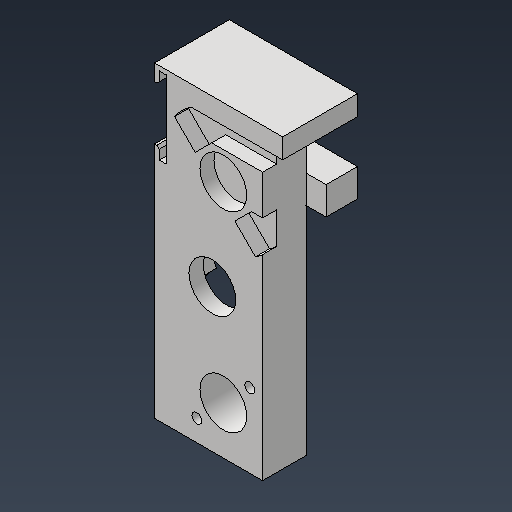
# Autodesk Inventor part: LeftGearbox
Saved by Autodesk Inventor 2026.2 (Build 302298010, 298A)
## iProperties
Created: 2026-04-13
Part Number: LeftGearbox
Material: Generic
Document SubType Name: Modeling
Designer: szymo
Density: 1 g/cm^3
Appearance: Default
Author: szymo
Autodesk Inventor part; units mm, degrees
ref_plane "YZ Plane" through (0, 0, 0) normal (1, 0, 0) x (0, 1, 0)
ref_plane "XZ Plane" through (0, 0, 0) normal (0, 1, 0) x (-1, 0, 0)
ref_plane "XY Plane" through (0, 0, 0) normal (0, 0, 1) x (1, 0, 0)
sketch "Sketch1" plane through (0, 0, 0) normal (0, 0, 1) x (1, 0, 0)
  circle A0 centre (14.7, -55.6371) radius 14.7 construction
  circle A1 centre (14.7, -55.6371) radius 14 construction
  circle A2 centre (14.7, -55.6371) radius 5
  circle A3 centre (14.7, -14.7) radius 5
  circle A4 centre (14.7, -14.7) radius 14 construction
  circle A5 centre (14.7, -14.7) radius 14.7 construction
  circle A6 centre (12.35, -35.2722) radius 5
  circle A7 centre (9.002, -47.4193) radius 8 construction
  circle A8 centre (9.002, -47.4193) radius 4.2 construction
  circle A9 centre (12.35, -35.2722) radius 9.6 construction
  line L0 (23.1, -65.8371) -> (0, -65.8371)
  line L1 (0, -65.8371) -> (0, 0)
  line L2 (0, 0) -> (23.1, 0)
  line L3 (23.1, 0) -> (23.1, -65.8371)
  circle A10 centre (12.35, -35.2722) radius 10
  circle A11 centre (9.002, -47.4193) radius 8.4
  line L4 (29.4, -55.6371) -> (23.1, -55.6371)
  line L5 (14.7, -55.6371) -> (23.1, -55.6371) construction
  line L6 (20.7104, -17.1749) -> (25.128, -21.5925) construction
  arc A12 (21.5925, -25.128) -> (25.128, -21.5925) centre (14.7, -14.7) ccw construction
  line L7 (21.5925, -25.128) -> (17.1749, -20.7104)
  arc A13 (17.1749, -20.7104) -> (20.7104, -17.1749) centre (14.7, -14.7) ccw construction
  arc A14 (7.8075, -4.272) -> (4.272, -7.8075) centre (14.7, -14.7) ccw
  line L8 (4.272, -7.8075) -> (8.6896, -12.2251)
  arc A15 (12.2251, -8.6896) -> (8.6896, -12.2251) centre (14.7, -14.7) ccw construction
  line L9 (12.2251, -8.6896) -> (7.8075, -4.272) construction
  line L10 (7.8075, -4.272) -> (23.1, -4.272)
  line L11 (12.2251, -8.6896) -> (23.1, -8.6896)
  line L12 (12.2251, -8.6896) -> (8.6896, -12.2251)
  line L13 (21.5925, -25.128) -> (23.1, -25.128)
  line L14 (20.7104, -17.1749) -> (23.1, -17.1749)
  line L15 (20.7104, -17.1749) -> (17.1749, -20.7104)
  line L16 (23.1, -4.272) -> (27.4, -4.272)
  line L17 (27.4, -4.272) -> (27.4, 0)
  line L18 (27.4, 0) -> (23.1, 0)
  circle A16 centre (9.002, -47.4193) radius 4.6
  circle A17 centre (14.7, -55.6371) radius 14.7 projected
  circle A18 centre (14.7, -55.6371) radius 14 projected
  circle A19 centre (9.0431, -61.2939) radius 1.0564 projected
  circle A20 centre (20.3569, -49.9802) radius 1.0564 projected
  circle A21 centre (14.7, -55.6371) radius 5 projected
  circle A22 centre (14.7, -55.6371) radius 14 projected
  circle A23 centre (14.7, -14.7) radius 14.7 projected
  circle A24 centre (14.7, -14.7) radius 14 projected
  line L19 (18.8355, -20.9568) -> (21.7016, -23.8229) projected
  arc A25 (21.7016, -23.8229) -> (23.8229, -21.7016) centre (14.7, -14.7) ccw projected
  line L20 (23.8229, -21.7016) -> (20.9568, -18.8355) projected
  arc A26 (18.8355, -20.9568) -> (20.9568, -18.8355) centre (14.7, -14.7) ccw projected
  arc A27 (7.6984, -5.5771) -> (5.5771, -7.6984) centre (14.7, -14.7) ccw projected
  line L21 (5.5771, -7.6984) -> (8.4432, -10.5645) projected
  arc A28 (10.5645, -8.4432) -> (8.4432, -10.5645) centre (14.7, -14.7) ccw projected
  line L22 (10.5645, -8.4432) -> (7.6984, -5.5771) projected
  circle A29 centre (14.7, -14.7) radius 5 projected
  circle A30 centre (14.7, -14.7) radius 14 projected
  arc A31 (9.8338, -26.0078) -> (9.7739, -27.4347) centre (15.759, -26.9712) ccw projected
  arc A32 (10.3221, -25.8888) -> (9.8338, -26.0078) centre (12.35, -35.2722) ccw projected
  arc A33 (11.0317, -27.1282) -> (10.3221, -25.8888) centre (5.5043, -29.47) ccw projected
  arc A34 (11.4597, -27.0704) -> (11.0317, -27.1282) centre (12.35, -35.2722) ccw projected
  arc A35 (11.815, -25.6871) -> (11.4597, -27.0704) centre (17.4104, -27.8613) ccw projected
  arc A36 (12.3173, -25.6723) -> (11.815, -25.6871) centre (12.35, -35.2722) ccw projected
  arc A37 (12.7537, -27.0321) -> (12.3173, -25.6723) centre (6.8602, -28.1735) ccw projected
  arc A38 (13.1844, -27.0645) -> (12.7537, -27.0321) centre (12.35, -35.2722) ccw projected
  arc A39 (13.8195, -25.7853) -> (13.1844, -27.0645) centre (18.8407, -29.0754) ccw projected
  arc A40 (14.314, -25.8753) -> (13.8195, -25.7853) centre (12.35, -35.2722) ccw projected
  arc A41 (14.4581, -27.2961) -> (14.314, -25.8753) centre (8.4561, -27.1873) ccw projected
  arc A42 (14.8727, -27.4174) -> (14.4581, -27.2961) centre (12.35, -35.2722) ccw projected
  arc A43 (15.7598, -26.2982) -> (14.8727, -27.4174) centre (19.9872, -30.5603) ccw projected
  arc A44 (16.2248, -26.4889) -> (15.7598, -26.2982) centre (12.35, -35.2722) ccw projected
  arc A45 (16.0704, -27.9087) -> (16.2248, -26.4889) centre (10.2221, -26.5543) ccw projected
  arc A46 (16.4507, -28.1135) -> (16.0704, -27.9087) centre (12.35, -35.2722) ccw projected
  arc A47 (17.5511, -27.2032) -> (16.4507, -28.1135) centre (20.8, -32.2511) ccw projected
  arc A48 (17.9663, -27.4865) -> (17.5511, -27.2032) centre (12.35, -35.2722) ccw projected
  arc A49 (17.52, -28.8431) -> (17.9663, -27.4865) centre (12.0812, -26.3024) ccw projected
  arc A50 (17.8494, -29.1225) -> (17.52, -28.8431) centre (12.35, -35.2722) ccw projected
  arc A51 (19.1151, -28.4609) -> (17.8494, -29.1225) centre (21.2434, -34.074) ccw projected
  arc A52 (19.4623, -28.8243) -> (19.1151, -28.4609) centre (12.35, -35.2722) ccw projected
  arc A53 (18.7437, -30.0585) -> (19.4623, -28.8243) centre (13.952, -26.4426) ccw projected
  arc A54 (19.0078, -30.4003) -> (18.7437, -30.0585) centre (12.35, -35.2722) ccw projected
  arc A55 (20.3834, -30.0163) -> (19.0078, -30.4003) centre (21.2982, -35.9492) ccw projected
  arc A56 (20.6475, -30.4439) -> (20.3834, -30.0163) centre (12.35, -35.2722) ccw projected
  arc A57 (19.688, -31.5018) -> (20.6475, -30.4439) centre (15.7527, -26.9686) ccw projected
  arc A58 (19.8753, -31.891) -> (19.688, -31.5018) centre (12.35, -35.2722) ccw projected
  arc A59 (21.3006, -31.8014) -> (19.8753, -31.891) centre (20.9619, -37.7949) ccw projected
  arc A60 (21.47, -32.2746) -> (21.3006, -31.8014) centre (12.35, -35.2722) ccw projected
  arc A61 (20.3116, -33.1099) -> (21.47, -32.2746) centre (17.4048, -27.8575) ccw projected
  arc A62 (20.4138, -33.5295) -> (20.3116, -33.1099) centre (12.35, -35.2722) ccw projected
  arc A63 (21.8266, -33.7382) -> (20.4138, -33.5295) centre (20.2492, -39.5303) ccw projected
  arc A64 (21.8939, -34.2363) -> (21.8266, -33.7382) centre (12.35, -35.2722) ccw projected
  arc A65 (20.5872, -34.8124) -> (21.8939, -34.2363) centre (18.836, -29.0705) ccw projected
  arc A66 (20.6, -35.2441) -> (20.5872, -34.8124) centre (12.35, -35.2722) ccw projected
  arc A67 (21.9385, -35.742) -> (20.6, -35.2441) centre (19.1913, -41.0796) ccw projected
  arc A68 (21.9008, -36.2432) -> (21.9385, -35.742) centre (12.35, -35.2722) ccw projected
  arc A69 (20.5028, -36.5351) -> (21.9008, -36.2432) centre (19.9836, -30.5545) ccw projected
  arc A70 (20.4255, -36.96) -> (20.5028, -36.5351) centre (12.35, -35.2722) ccw projected
  arc A71 (21.6313, -37.7253) -> (20.4255, -36.96) centre (17.8344, -42.3751) ccw projected
  arc A72 (21.4902, -38.2077) -> (21.6313, -37.7253) centre (12.35, -35.2722) ccw projected
  arc A73 (20.0621, -38.2025) -> (21.4902, -38.2077) centre (20.7977, -32.2447) ccw projected
  arc A74 (19.8981, -38.6021) -> (20.0621, -38.2025) centre (12.35, -35.2722) ccw projected
  arc A75 (20.9184, -39.6014) -> (19.8981, -38.6021) centre (16.2378, -43.3601) ccw projected
  arc A76 (20.6801, -40.0439) -> (20.9184, -39.6014) centre (12.35, -35.2722) ccw projected
  arc A77 (19.2843, -39.7419) -> (20.6801, -40.0439) centre (21.2425, -34.0672) ccw projected
  arc A78 (19.0409, -40.0987) -> (19.2843, -39.7419) centre (12.35, -35.2722) ccw projected
  arc A79 (19.8311, -41.2883) -> (19.0409, -40.0987) centre (14.4713, -43.9917) ccw projected
  arc A80 (19.506, -41.6716) -> (19.8311, -41.2883) centre (12.35, -35.2722) ccw projected
  arc A81 (18.2034, -41.086) -> (19.506, -41.6716) centre (21.2987, -35.9424) ccw projected
  arc A82 (17.8912, -41.3843) -> (18.2034, -41.086) centre (12.35, -35.2722) ccw projected
  arc A83 (18.4168, -42.7122) -> (17.8912, -41.3843) centre (12.612, -44.2422) ccw projected
  arc A84 (18.0191, -43.0195) -> (18.4168, -42.7122) centre (12.35, -35.2722) ccw projected
  arc A85 (16.8668, -42.1759) -> (18.0191, -43.0195) centre (20.9638, -37.7883) ccw projected
  arc A86 (16.4993, -42.4028) -> (16.8668, -42.1759) centre (12.35, -35.2722) ccw projected
  arc A87 (16.7374, -43.811) -> (16.4993, -42.4028) centre (10.7413, -44.1007) ccw projected
  arc A88 (16.2845, -44.0289) -> (16.7374, -43.811) centre (12.35, -35.2722) ccw projected
  arc A89 (15.3327, -42.9641) -> (16.2845, -44.0289) centre (20.2525, -39.5243) ccw projected
  arc A90 (14.9261, -43.1097) -> (15.3327, -42.9641) centre (12.35, -35.2722) ccw projected
  arc A91 (14.8662, -44.5366) -> (14.9261, -43.1097) centre (8.941, -43.5733) ccw projected
  arc A92 (14.3779, -44.6556) -> (14.8662, -44.5366) centre (12.35, -35.2722) ccw projected
  arc A93 (13.6683, -43.4162) -> (14.3779, -44.6556) centre (19.1957, -41.0744) ccw projected
  arc A94 (13.2403, -43.474) -> (13.6683, -43.4162) centre (12.35, -35.2722) ccw projected
  arc A95 (12.885, -44.8573) -> (13.2403, -43.474) centre (7.2896, -42.6831) ccw projected
  arc A96 (12.3827, -44.8722) -> (12.885, -44.8573) centre (12.35, -35.2722) ccw projected
  arc A97 (11.9463, -43.5123) -> (12.3827, -44.8722) centre (17.8398, -42.3709) ccw projected
  arc A98 (11.5156, -43.4799) -> (11.9463, -43.5123) centre (12.35, -35.2722) ccw projected
  arc A99 (10.8805, -44.7591) -> (11.5156, -43.4799) centre (5.8593, -41.469) ccw projected
  arc A100 (10.386, -44.6692) -> (10.8805, -44.7591) centre (12.35, -35.2722) ccw projected
  arc A101 (10.2419, -43.2483) -> (10.386, -44.6692) centre (16.2439, -43.3572) ccw projected
  arc A102 (9.8273, -43.1271) -> (10.2419, -43.2483) centre (12.35, -35.2722) ccw projected
  arc A103 (8.9402, -44.2462) -> (9.8273, -43.1271) centre (4.7128, -39.9841) ccw projected
  arc A104 (8.4752, -44.0555) -> (8.9402, -44.2462) centre (12.35, -35.2722) ccw projected
  arc A105 (8.6296, -42.6357) -> (8.4752, -44.0555) centre (14.4779, -43.9901) ccw projected
  arc A106 (8.2493, -42.4309) -> (8.6296, -42.6357) centre (12.35, -35.2722) ccw projected
  arc A107 (7.1489, -43.3412) -> (8.2493, -42.4309) centre (3.9, -38.2933) ccw projected
  arc A108 (6.7337, -43.0579) -> (7.1489, -43.3412) centre (12.35, -35.2722) ccw projected
  arc A109 (7.18, -41.7013) -> (6.7337, -43.0579) centre (12.6188, -44.242) ccw projected
  arc A110 (6.8506, -41.4219) -> (7.18, -41.7013) centre (12.35, -35.2722) ccw projected
  arc A111 (5.5849, -42.0835) -> (6.8506, -41.4219) centre (3.4566, -36.4704) ccw projected
  arc A112 (5.2377, -41.7201) -> (5.5849, -42.0835) centre (12.35, -35.2722) ccw projected
  arc A113 (5.9563, -40.4859) -> (5.2377, -41.7201) centre (10.748, -44.1019) ccw projected
  arc A114 (5.6922, -40.1441) -> (5.9563, -40.4859) centre (12.35, -35.2722) ccw projected
  arc A115 (4.3166, -40.5281) -> (5.6922, -40.1441) centre (3.4018, -34.5952) ccw projected
  arc A116 (4.0525, -40.1005) -> (4.3166, -40.5281) centre (12.35, -35.2722) ccw projected
  arc A117 (5.012, -39.0426) -> (4.0525, -40.1005) centre (8.9473, -43.5759) ccw projected
  arc A118 (4.8247, -38.6534) -> (5.012, -39.0426) centre (12.35, -35.2722) ccw projected
  arc A119 (3.3994, -38.743) -> (4.8247, -38.6534) centre (3.7381, -32.7495) ccw projected
  arc A120 (3.23, -38.2698) -> (3.3994, -38.743) centre (12.35, -35.2722) ccw projected
  arc A121 (4.3884, -37.4346) -> (3.23, -38.2698) centre (7.2952, -42.6869) ccw projected
  arc A122 (4.2862, -37.0149) -> (4.3884, -37.4346) centre (12.35, -35.2722) ccw projected
  arc A123 (2.8734, -36.8062) -> (4.2862, -37.0149) centre (4.4508, -31.0141) ccw projected
  arc A124 (2.8061, -36.3082) -> (2.8734, -36.8062) centre (12.35, -35.2722) ccw projected
  arc A125 (4.1128, -35.732) -> (2.8061, -36.3082) centre (5.864, -41.474) ccw projected
  arc A126 (4.1, -35.3003) -> (4.1128, -35.732) centre (12.35, -35.2722) ccw projected
  arc A127 (2.7615, -34.8024) -> (4.1, -35.3003) centre (5.5087, -29.4648) ccw projected
  arc A128 (2.7992, -34.3012) -> (2.7615, -34.8024) centre (12.35, -35.2722) ccw projected
  arc A129 (4.1972, -34.0094) -> (2.7992, -34.3012) centre (4.7164, -39.9899) ccw projected
  arc A130 (4.2745, -33.5844) -> (4.1972, -34.0094) centre (12.35, -35.2722) ccw projected
  arc A131 (3.0687, -32.8191) -> (4.2745, -33.5844) centre (6.8656, -28.1694) ccw projected
  arc A132 (3.2098, -32.3367) -> (3.0687, -32.8191) centre (12.35, -35.2722) ccw projected
  arc A133 (4.6379, -32.3419) -> (3.2098, -32.3367) centre (3.9023, -38.2997) ccw projected
  arc A134 (4.8019, -31.9423) -> (4.6379, -32.3419) centre (12.35, -35.2722) ccw projected
  arc A135 (3.7816, -30.943) -> (4.8019, -31.9423) centre (8.4622, -27.1843) ccw projected
  arc A136 (4.0199, -30.5005) -> (3.7816, -30.943) centre (12.35, -35.2722) ccw projected
  arc A137 (5.4157, -30.8025) -> (4.0199, -30.5005) centre (3.4575, -36.4772) ccw projected
  arc A138 (5.6591, -30.4457) -> (5.4157, -30.8025) centre (12.35, -35.2722) ccw projected
  arc A139 (4.8689, -29.2562) -> (5.6591, -30.4457) centre (10.2287, -26.5527) ccw projected
  arc A140 (5.194, -28.8729) -> (4.8689, -29.2562) centre (12.35, -35.2722) ccw projected
  arc A141 (6.4966, -29.4585) -> (5.194, -28.8729) centre (3.4013, -34.602) ccw projected
  arc A142 (6.8088, -29.1601) -> (6.4966, -29.4585) centre (12.35, -35.2722) ccw projected
  arc A143 (6.2832, -27.8322) -> (6.8088, -29.1601) centre (12.088, -26.3022) ccw projected
  arc A144 (6.6809, -27.5249) -> (6.2832, -27.8322) centre (12.35, -35.2722) ccw projected
  arc A145 (7.8332, -28.3685) -> (6.6809, -27.5249) centre (3.7362, -32.7561) ccw projected
  arc A146 (8.2007, -28.1416) -> (7.8332, -28.3685) centre (12.35, -35.2722) ccw projected
  arc A147 (7.9626, -26.7334) -> (8.2007, -28.1416) centre (13.9587, -26.4438) ccw projected
  arc A148 (8.4155, -26.5155) -> (7.9626, -26.7334) centre (12.35, -35.2722) ccw projected
  arc A149 (9.3673, -27.5803) -> (8.4155, -26.5155) centre (4.4475, -31.0201) ccw projected
  arc A150 (9.7739, -27.4347) -> (9.3673, -27.5803) centre (12.35, -35.2722) ccw projected
  circle A151 centre (9.002, -47.4193) radius 1.25 projected
  arc A152 (9.3068, -54.2875) -> (9.7745, -55.3819) centre (14.1081, -52.8828) ccw projected
  arc A153 (8.9469, -54.294) -> (9.3068, -54.2875) centre (9.002, -47.4193) ccw projected
  arc A154 (8.5194, -55.4047) -> (8.9469, -54.294) centre (4.0978, -53.0648) ccw projected
  arc A155 (8.1021, -55.3685) -> (8.5194, -55.4047) centre (9.002, -47.4193) ccw projected
  arc A156 (7.8722, -54.2008) -> (8.1021, -55.3685) centre (12.8606, -53.8251) ccw projected
  arc A157 (7.5188, -54.1324) -> (7.8722, -54.2008) centre (9.002, -47.4193) ccw projected
  arc A158 (6.8696, -55.1298) -> (7.5188, -54.1324) centre (3.0312, -51.9218) ccw projected
  arc A159 (6.469, -55.0077) -> (6.8696, -55.1298) centre (9.002, -47.4193) ccw projected
  arc A160 (6.4869, -53.8177) -> (6.469, -55.0077) centre (11.4444, -54.4873) ccw projected
  arc A161 (6.1555, -53.6773) -> (6.4869, -53.8177) centre (9.002, -47.4193) ccw projected
  arc A162 (5.3131, -54.518) -> (6.1555, -53.6773) centre (2.2255, -50.582) ccw projected
  arc A163 (4.9466, -54.3152) -> (5.3131, -54.518) centre (9.002, -47.4193) ccw projected
  arc A164 (5.2115, -53.155) -> (4.9466, -54.3152) centre (9.9215, -54.8407) ccw projected
  arc A165 (4.9166, -52.9487) -> (5.2115, -53.155) centre (9.002, -47.4193) ccw projected
  arc A166 (3.9178, -53.5959) -> (4.9166, -52.9487) centre (1.716, -49.104) ccw projected
  arc A167 (3.6015, -53.3214) -> (3.9178, -53.5959) centre (9.002, -47.4193) ccw projected
  arc A168 (4.1019, -52.2416) -> (3.6015, -53.3214) centre (8.3584, -54.8697) ccw projected
  arc A169 (3.8562, -51.9785) -> (4.1019, -52.2416) centre (9.002, -47.4193) ccw projected
  arc A170 (2.7447, -52.4039) -> (3.8562, -51.9785) centre (1.525, -47.5523) ccw projected
  arc A171 (2.4924, -52.0696) -> (2.7447, -52.4039) centre (9.002, -47.4193) ccw projected
  arc A172 (3.2063, -51.1174) -> (2.4924, -52.0696) centre (6.8235, -54.5731) ccw projected
  arc A173 (3.0207, -50.809) -> (3.2063, -51.1174) centre (9.002, -47.4193) ccw projected
  arc A174 (1.8451, -50.994) -> (3.0207, -50.809) centre (1.6607, -45.9949) ccw projected
  arc A175 (1.6678, -50.6146) -> (1.8451, -50.994) centre (9.002, -47.4193) ccw projected
  arc A176 (2.5641, -49.8316) -> (1.6678, -50.6146) centre (5.3837, -53.9638) ccw projected
  arc A177 (2.4467, -49.4913) -> (2.5641, -49.8316) centre (9.002, -47.4193) ccw projected
  arc A178 (1.2582, -49.4279) -> (2.4467, -49.4913) centre (2.1173, -44.4997) ccw projected
  arc A179 (1.1637, -49.0199) -> (1.2582, -49.4279) centre (9.002, -47.4193) ccw projected
  arc A180 (2.2032, -48.4404) -> (1.1637, -49.0199) centre (4.1021, -53.0685) ccw projected
  arc A181 (2.1591, -48.0831) -> (2.2032, -48.4404) centre (9.002, -47.4193) ccw projected
  arc A182 (1.0098, -47.774) -> (2.1591, -48.0831) centre (2.8747, -43.1321) ccw projected
  arc A183 (1.0022, -47.3552) -> (1.0098, -47.774) centre (9.002, -47.4193) ccw projected
  arc A184 (2.1395, -47.0045) -> (1.0022, -47.3552) centre (3.0346, -51.9263) ccw projected
  arc A185 (2.1706, -46.6459) -> (2.1395, -47.0045) centre (9.002, -47.4193) ccw projected
  arc A186 (1.1107, -46.1046) -> (2.1706, -46.6459) centre (3.9, -41.9518) ccw projected
  arc A187 (1.1904, -45.6934) -> (1.1107, -46.1046) centre (9.002, -47.4193) ccw projected
  arc A188 (2.3757, -45.5868) -> (1.1904, -45.6934) centre (2.2279, -50.5871) ccw projected
  arc A189 (2.4807, -45.2425) -> (2.3757, -45.5868) centre (9.002, -47.4193) ccw projected
  arc A190 (1.5565, -44.4926) -> (2.4807, -45.2425) centre (5.1482, -41.0105) ccw projected
  arc A191 (1.7199, -44.107) -> (1.5565, -44.4926) centre (9.002, -47.4193) ccw projected
  arc A192 (2.9015, -44.2491) -> (1.7199, -44.107) centre (1.7173, -49.1095) ccw projected
  arc A193 (3.0758, -43.9342) -> (2.9015, -44.2491) centre (9.002, -47.4193) ccw projected
  arc A194 (2.3277, -43.0086) -> (3.0758, -43.9342) centre (6.5649, -40.3493) ccw projected
  arc A195 (2.5677, -42.6653) -> (2.3277, -43.0086) centre (9.002, -47.4193) ccw projected
  arc A196 (3.6939, -43.0501) -> (2.5677, -42.6653) centre (1.5251, -47.558) ccw projected
  arc A197 (3.9298, -42.7782) -> (3.6939, -43.0501) centre (9.002, -47.4193) ccw projected
  arc A198 (3.3906, -41.7173) -> (3.9298, -42.7782) centre (8.0881, -39.9971) ccw projected
  arc A199 (3.6967, -41.4314) -> (3.3906, -41.7173) centre (9.002, -47.4193) ccw projected
  arc A200 (4.7183, -42.0419) -> (3.6967, -41.4314) centre (1.6596, -46.0004) ccw projected
  arc A201 (5.0056, -41.8251) -> (4.7183, -42.0419) centre (9.002, -47.4193) ccw projected
  arc A202 (4.6987, -40.6752) -> (5.0056, -41.8251) centre (9.6512, -39.9693) ccw projected
  arc A203 (5.0576, -40.4593) -> (4.6987, -40.6752) centre (9.002, -47.4193) ccw projected
  arc A204 (5.9299, -41.2688) -> (5.0576, -40.4593) centre (2.1151, -44.5049) ccw projected
  arc A205 (6.256, -41.1165) -> (5.9299, -41.2688) centre (9.002, -47.4193) ccw projected
  arc A206 (6.1949, -39.9279) -> (6.256, -41.1165) centre (11.1859, -40.2671) ccw projected
  arc A207 (6.5908, -39.7913) -> (6.1949, -39.9279) centre (9.002, -47.4193) ccw projected
  arc A208 (7.2758, -40.7645) -> (6.5908, -39.7913) centre (2.8715, -43.1367) ccw projected
  arc A209 (7.6264, -40.6833) -> (7.2758, -40.7645) centre (9.002, -47.4193) ccw projected
  arc A210 (7.8138, -39.508) -> (7.6264, -40.6833) centre (12.6252, -40.8775) ccw projected
  arc A211 (8.2295, -39.4566) -> (7.8138, -39.508) centre (9.002, -47.4193) ccw projected
  arc A212 (8.6971, -40.551) -> (8.2295, -39.4566) centre (3.8958, -41.9557) ccw projected
  arc A213 (9.057, -40.5445) -> (8.6971, -40.551) centre (9.002, -47.4193) ccw projected
  arc A214 (9.4846, -39.4338) -> (9.057, -40.5445) centre (13.9062, -41.7737) ccw projected
  arc A215 (9.9019, -39.47) -> (9.4846, -39.4338) centre (9.002, -47.4193) ccw projected
  arc A216 (10.1318, -40.6377) -> (9.9019, -39.47) centre (5.1434, -41.0135) ccw projected
  arc A217 (10.4851, -40.7061) -> (10.1318, -40.6377) centre (9.002, -47.4193) ccw projected
  arc A218 (11.1343, -39.7087) -> (10.4851, -40.7061) centre (14.9728, -42.9167) ccw projected
  arc A219 (11.5349, -39.8308) -> (11.1343, -39.7087) centre (9.002, -47.4193) ccw projected
  arc A220 (11.517, -41.0208) -> (11.5349, -39.8308) centre (6.5595, -40.3512) ccw projected
  arc A221 (11.8485, -41.1612) -> (11.517, -41.0208) centre (9.002, -47.4193) ccw projected
  arc A222 (12.6908, -40.3205) -> (11.8485, -41.1612) centre (15.7784, -44.2565) ccw projected
  arc A223 (13.0573, -40.5233) -> (12.6908, -40.3205) centre (9.002, -47.4193) ccw projected
  arc A224 (12.7924, -41.6836) -> (13.0573, -40.5233) centre (8.0824, -39.9978) ccw projected
  arc A225 (13.0874, -41.8898) -> (12.7924, -41.6836) centre (9.002, -47.4193) ccw projected
  arc A226 (14.0861, -41.2426) -> (13.0874, -41.8898) centre (16.2879, -45.7345) ccw projected
  arc A227 (14.4024, -41.5171) -> (14.0861, -41.2426) centre (9.002, -47.4193) ccw projected
  arc A228 (13.9021, -42.597) -> (14.4024, -41.5171) centre (9.6455, -39.9688) ccw projected
  arc A229 (14.1477, -42.86) -> (13.9021, -42.597) centre (9.002, -47.4193) ccw projected
  arc A230 (15.2592, -42.4346) -> (14.1477, -42.86) centre (16.479, -47.2862) ccw projected
  arc A231 (15.5115, -42.7689) -> (15.2592, -42.4346) centre (9.002, -47.4193) ccw projected
  arc A232 (14.7976, -43.7211) -> (15.5115, -42.7689) centre (11.1805, -40.2654) ccw projected
  arc A233 (14.9832, -44.0295) -> (14.7976, -43.7211) centre (9.002, -47.4193) ccw projected
  arc A234 (16.1589, -43.8445) -> (14.9832, -44.0295) centre (16.3432, -48.8436) ccw projected
  arc A235 (16.3361, -44.224) -> (16.1589, -43.8445) centre (9.002, -47.4193) ccw projected
  arc A236 (15.4399, -45.0069) -> (16.3361, -44.224) centre (12.6202, -40.8747) ccw projected
  arc A237 (15.5573, -45.3472) -> (15.4399, -45.0069) centre (9.002, -47.4193) ccw projected
  arc A238 (16.7457, -45.4106) -> (15.5573, -45.3472) centre (15.8867, -50.3389) ccw projected
  arc A239 (16.8402, -45.8187) -> (16.7457, -45.4106) centre (9.002, -47.4193) ccw projected
  arc A240 (15.8007, -46.3982) -> (16.8402, -45.8187) centre (13.9019, -41.77) ccw projected
  arc A241 (15.8448, -46.7554) -> (15.8007, -46.3982) centre (9.002, -47.4193) ccw projected
  arc A242 (16.9941, -47.0645) -> (15.8448, -46.7554) centre (15.1292, -51.7065) ccw projected
  arc A243 (17.0017, -47.4833) -> (16.9941, -47.0645) centre (9.002, -47.4193) ccw projected
  arc A244 (15.8644, -47.834) -> (17.0017, -47.4833) centre (14.9693, -42.9122) ccw projected
  arc A245 (15.8333, -48.1926) -> (15.8644, -47.834) centre (9.002, -47.4193) ccw projected
  arc A246 (16.8932, -48.7339) -> (15.8333, -48.1926) centre (14.1039, -52.8867) ccw projected
  arc A247 (16.8136, -49.1451) -> (16.8932, -48.7339) centre (9.002, -47.4193) ccw projected
  arc A248 (15.6283, -49.2517) -> (16.8136, -49.1451) centre (15.776, -44.2514) ccw projected
  arc A249 (15.5233, -49.596) -> (15.6283, -49.2517) centre (9.002, -47.4193) ccw projected
  arc A250 (16.4474, -50.3459) -> (15.5233, -49.596) centre (12.8557, -53.828) ccw projected
  arc A251 (16.2841, -50.7315) -> (16.4474, -50.3459) centre (9.002, -47.4193) ccw projected
  arc A252 (15.1025, -50.5894) -> (16.2841, -50.7315) centre (16.2866, -45.729) ccw projected
  arc A253 (14.9282, -50.9043) -> (15.1025, -50.5894) centre (9.002, -47.4193) ccw projected
  arc A254 (15.6762, -51.8299) -> (14.9282, -50.9043) centre (11.439, -54.4892) ccw projected
  arc A255 (15.4363, -52.1732) -> (15.6762, -51.8299) centre (9.002, -47.4193) ccw projected
  arc A256 (14.31, -51.7885) -> (15.4363, -52.1732) centre (16.4789, -47.2805) ccw projected
  arc A257 (14.0741, -52.0603) -> (14.31, -51.7885) centre (9.002, -47.4193) ccw projected
  arc A258 (14.6134, -53.1212) -> (14.0741, -52.0603) centre (9.9159, -54.8414) ccw projected
  arc A259 (14.3073, -53.4071) -> (14.6134, -53.1212) centre (9.002, -47.4193) ccw projected
  arc A260 (13.2856, -52.7966) -> (14.3073, -53.4071) centre (16.3443, -48.8381) ccw projected
  arc A261 (12.9983, -53.0134) -> (13.2856, -52.7966) centre (9.002, -47.4193) ccw projected
  arc A262 (13.3052, -54.1633) -> (12.9983, -53.0134) centre (8.3528, -54.8692) ccw projected
  arc A263 (12.9464, -54.3793) -> (13.3052, -54.1633) centre (9.002, -47.4193) ccw projected
  arc A264 (12.074, -53.5697) -> (12.9464, -54.3793) centre (15.8889, -50.3336) ccw projected
  arc A265 (11.7479, -53.7221) -> (12.074, -53.5697) centre (9.002, -47.4193) ccw projected
  arc A266 (11.809, -54.9106) -> (11.7479, -53.7221) centre (6.818, -54.5714) ccw projected
  arc A267 (11.4131, -55.0473) -> (11.809, -54.9106) centre (9.002, -47.4193) ccw projected
  arc A268 (10.7281, -54.074) -> (11.4131, -55.0473) centre (15.1325, -51.7018) ccw projected
  arc A269 (10.3775, -54.1552) -> (10.7281, -54.074) centre (9.002, -47.4193) ccw projected
  arc A270 (10.1902, -55.3305) -> (10.3775, -54.1552) centre (5.3787, -53.9611) ccw projected
  arc A271 (9.7745, -55.3819) -> (10.1902, -55.3305) centre (9.002, -47.4193) ccw projected
  circle A272 centre (9.002, -47.4193) radius 1.25 projected
  arc A273 (10.0792, -44.7807) -> (10.0684, -43.3569) centre (6.4384, -44.0965) ccw projected
  arc A274 (10.4144, -44.9439) -> (10.0792, -44.7807) centre (9.002, -47.4193) ccw projected
  arc A275 (11.5418, -44.0742) -> (10.4144, -44.9439) centre (13.1986, -47.3876) ccw projected
  arc A276 (11.9567, -44.4343) -> (11.5418, -44.0742) centre (9.002, -47.4193) ccw projected
  arc A277 (11.2542, -45.6728) -> (11.9567, -44.4343) centre (8.4432, -43.2599) ccw projected
  arc A278 (11.4629, -45.9817) -> (11.2542, -45.6728) centre (9.002, -47.4193) ccw projected
  arc A279 (12.874, -45.7923) -> (11.4629, -45.9817) centre (12.6522, -49.4902) ccw projected
  arc A280 (13.0533, -46.3116) -> (12.874, -45.7923) centre (9.002, -47.4193) ccw projected
  arc A281 (11.8257, -47.0329) -> (13.0533, -46.3116) centre (10.5978, -43.5377) ccw projected
  arc A282 (11.8519, -47.4048) -> (11.8257, -47.0329) centre (9.002, -47.4193) ccw projected
  arc A283 (13.1688, -47.9463) -> (11.8519, -47.4048) centre (11.1277, -51.0378) ccw projected
  arc A284 (13.0643, -48.4857) -> (13.1688, -47.9463) centre (9.002, -47.4193) ccw projected
  arc A285 (11.6405, -48.4965) -> (13.0643, -48.4857) centre (12.3247, -44.8557) ccw projected
  arc A286 (11.4774, -48.8317) -> (11.6405, -48.4965) centre (9.002, -47.4193) ccw projected
  arc A287 (12.347, -49.9591) -> (11.4774, -48.8317) centre (9.0336, -51.6159) ccw projected
  arc A288 (11.9869, -50.374) -> (12.347, -49.9591) centre (9.002, -47.4193) ccw projected
  arc A289 (10.7484, -49.6715) -> (11.9869, -50.374) centre (13.1614, -46.8605) ccw projected
  arc A290 (10.4395, -49.8802) -> (10.7484, -49.6715) centre (9.002, -47.4193) ccw projected
  arc A291 (10.629, -51.2913) -> (10.4395, -49.8802) centre (6.9311, -51.0695) ccw projected
  arc A292 (10.1096, -51.4706) -> (10.629, -51.2913) centre (9.002, -47.4193) ccw projected
  arc A293 (9.3883, -50.2429) -> (10.1096, -51.4706) centre (12.8835, -49.0151) ccw projected
  arc A294 (9.0165, -50.2692) -> (9.3883, -50.2429) centre (9.002, -47.4193) ccw projected
  arc A295 (8.4749, -51.5861) -> (9.0165, -50.2692) centre (5.3834, -49.545) ccw projected
  arc A296 (7.9356, -51.4816) -> (8.4749, -51.5861) centre (9.002, -47.4193) ccw projected
  arc A297 (7.9247, -50.0578) -> (7.9356, -51.4816) centre (11.5656, -50.742) ccw projected
  arc A298 (7.5895, -49.8946) -> (7.9247, -50.0578) centre (9.002, -47.4193) ccw projected
  arc A299 (6.4622, -50.7643) -> (7.5895, -49.8946) centre (4.8053, -47.4509) ccw projected
  arc A300 (6.0473, -50.4042) -> (6.4622, -50.7643) centre (9.002, -47.4193) ccw projected
  arc A301 (6.7498, -49.1657) -> (6.0473, -50.4042) centre (9.5607, -51.5786) ccw projected
  arc A302 (6.5411, -48.8568) -> (6.7498, -49.1657) centre (9.002, -47.4193) ccw projected
  arc A303 (5.1299, -49.0462) -> (6.5411, -48.8568) centre (5.3518, -45.3483) ccw projected
  arc A304 (4.9507, -48.5269) -> (5.1299, -49.0462) centre (9.002, -47.4193) ccw projected
  arc A305 (6.1783, -47.8056) -> (4.9507, -48.5269) centre (7.4062, -51.3008) ccw projected
  arc A306 (6.152, -47.4338) -> (6.1783, -47.8056) centre (9.002, -47.4193) ccw projected
  arc A307 (4.8352, -46.8922) -> (6.152, -47.4338) centre (6.8763, -43.8007) ccw projected
  arc A308 (4.9396, -46.3529) -> (4.8352, -46.8922) centre (9.002, -47.4193) ccw projected
  arc A309 (6.3634, -46.342) -> (4.9396, -46.3529) centre (5.6792, -49.9828) ccw projected
  arc A310 (6.5266, -46.0068) -> (6.3634, -46.342) centre (9.002, -47.4193) ccw projected
  arc A311 (5.6569, -44.8794) -> (6.5266, -46.0068) centre (8.9703, -43.2226) ccw projected
  arc A312 (6.0171, -44.4646) -> (5.6569, -44.8794) centre (9.002, -47.4193) ccw projected
  arc A313 (7.2555, -45.1671) -> (6.0171, -44.4646) centre (4.8426, -47.978) ccw projected
  arc A314 (7.5644, -44.9584) -> (7.2555, -45.1671) centre (9.002, -47.4193) ccw projected
  arc A315 (7.375, -43.5472) -> (7.5644, -44.9584) centre (11.0729, -43.7691) ccw projected
  arc A316 (7.8943, -43.368) -> (7.375, -43.5472) centre (9.002, -47.4193) ccw projected
  arc A317 (8.6156, -44.5956) -> (7.8943, -43.368) centre (5.1205, -45.8234) ccw projected
  arc A318 (8.9875, -44.5693) -> (8.6156, -44.5956) centre (9.002, -47.4193) ccw projected
  arc A319 (9.529, -43.2525) -> (8.9875, -44.5693) centre (12.6205, -45.2935) ccw projected
  arc A320 (10.0684, -43.3569) -> (9.529, -43.2525) centre (9.002, -47.4193) ccw projected
  circle A321 centre (12.35, -35.2722) radius 4.8 projected
  line L23 (2.5, -1) -> (1, -1)
  line L24 (1, -1) -> (1, -17.5)
  line L25 (1, -17.5) -> (2.5, -17.5)
  line L26 (2.5, -17.5) -> (2.5, -1)
  line L27 (1.5, -1) -> (1.5, -17) projected
  line L28 (2.5, -1) -> (1.5, -1) projected
  line L29 (2.5, -17) -> (2.5, -1) projected
  line L30 (2.5, -17) -> (1.5, -17) projected
  line L31 (1, -15) -> (0, -15)
  line L32 (1, -3.5) -> (0, -3.5)
  point P0 (0, 0)
  point P1 (3.9544, -40.7049)
  point P2 (16.7767, -44.2391)
  point P3 (13.2732, -40.1862)
  point P4 (9.0396, -39.0193)
  point P5 (13.0569, -45.2472)
  point P6 (6.6325, -43.4765)
  point P7 (16.5957, -51.0104)
  point P8 (9.7023, -55.79)
  point P9 (0.0031, -15)
  point P10 (0, -14.7)
  dimension "d0" = 4.5
  dimension "d2" = 0.4
  dimension "d3" = 0.4
  dimension "d5" = 6.3
  dimension "d8" = 2
  dimension "d10" = 0.4
  dimension "d19" = 10
  dimension "d20" = 1
  dimension "d21" = 1
  dimension "d22" = 1
  dimension "d24" = 1
  dimension "d25" = 1
  dimension "d26" = 1
  dimension "d27" = 1
  dimension "d28" = 1
  dimension "d56" = 0.5
  dimension "d57" = 0.5
  dimension "d77" = 2.5
  dimension "d78" = 2.5
  constraints: 50 end point, 13 centre point, 12 point on line, 11 perpendicular, 10 coincident, 8 point on circle, 5 parallel, 5 tangent, 2 horizontal, 2 horizontal alignment, 1 collinear, 17 other
  measures "d5" distance of L4.start L4.end
  measures "d8" distance edge to line of A5 L17
  measures "d19" diameter of A6
  measures "d20" distance between parallel lines of L7 L19
  measures "d21" radial gap between concentric circles of A12 A25
  measures "d22" radial gap between concentric circles of A13 A26
  measures "d24" distance between parallel lines of L6 L20
  measures "d25" distance between parallel lines of L9 L22
  measures "d26" distance between parallel lines of L8 L21
  measures "d27" radial gap between concentric circles of A28 A15
  measures "d28" radial gap between concentric circles of A14 A27
  measures "d56" distance between parallel lines of L24 L27
  measures "d57" distance between parallel lines of L25 L30
  measures "d77" distance between parallel lines of L28 L32
  measures "d78" distance between parallel lines of L25 L31
extrude "Extrusion1" add sketch "Sketch1" against normal blind 1.6 contours A2 A11 A10 A18 L3 L0 | A2 A253 A252 A251 A250 A249 A248 A247 A246 A245 A244 A243 A242 A241 A240 A239 A238 A237 A236 A10 A11 | A11 A18 A178 A177 A176 A175 A174 A173 A172 A171 A170 A169 A168 A167 A166 A165 A164 A163 A162 A161 A160 A159 A158 A157 A156 A155 A154 A153 A152 A2 | A2 A152 A153 A154 A155 A156 A157 A158 A159 A160 A161 A162 A163 A164 A165 A166 A167 A168 A169 A170 A171 A172 A173 A174 A175 A176 A177 A178 A18 A16 A10 A236 A237 A238 A239 A240 A241 A242 A243 A244 A245 A246 A247 A248 A249 A250 A251 A252 A253 | A18 L0 A17 A11 | A11 A17 A178 A18 | A11 A88 A87 A86 A85 A84 A83 A18 A10 | A10 A236 A235 A89 A88 A11 | A17 L1 L31 A23 A10 A11 | A11 A10 A201 A200 A199 A198 A197 A196 A195 A194 A193 A192 A191 A190 A189 A188 A187 A186 A185 A184 A183 A182 A17 A180 A179 A178 | A178 A17 A180 A181 A182 A10 A16 A18 | A10 A16 A96 A95 A94 A93 A92 A91 A233 A234 A89 A235 A236 | A18 A83 A82 A17 A10 | A10 A17 L3 A18 | A88 A89 A235 A234 A232 A231 A230 A229 A228 A18 A11 | A11 A18 A83 A84 A85 A86 A87 A88 | A11 A116 A115 A114 A113 A204 A203 A202 A201 A10 | A10 A23 A147 A146 A145 A144 A143 A142 A141 A140 A139 A138 A137 A136 A135 A134 A133 A132 A131 A130 A129 A128 A127 A126 A125 A124 A123 A122 A121 A120 A119 A118 A117 A116 A11 | A178 A179 A180 A17 | A17 L0 L1 | A18 A311 A310 A309 A308 A307 A306 A305 A304 A303 A302 A301 A300 A299 A298 A297 A296 A295 A294 A293 A292 A291 A290 A289 A288 A287 A286 A285 A284 A283 A282 A281 A280 A279 A278 A277 A10 A16 | A16 A10 A18 A313 A312 A311 | A10 A277 A276 A275 A99 A16 A97 A96 | A17 A82 A81 A80 A79 A78 A77 A76 A75 A74 A73 A72 A71 A70 A69 A68 A67 A66 A65 A64 A63 A62 A61 A60 A59 A58 A57 A56 A55 A54 A53 A52 A23 A10 | A10 A23 L3 A17 | A18 A11 A17 A82 A83 | A18 A228 A227 A226 A225 A224 A17 A11 | A23 L31 A24 A10 | A10 A24 A147 A23 | A201 A202 A203 A204 A113 A112 A111 A110 A109 A108 A17 A10 | A10 A17 A182 A183 A184 A185 A186 A187 A188 A189 A190 A191 A192 A193 A194 A195 A196 A197 A198 A199 A200 A201 | A116 A117 A118 A119 A120 A121 A122 A123 A124 A125 A126 A127 A128 A129 A130 A131 A132 A133 A134 A135 A136 A137 A138 A139 A140 A141 A142 A143 A144 A145 A146 A147 A23 A50 A51 A52 A53 A54 A55 A56 A57 A58 A59 A60 A61 A62 A63 A64 A65 A66 A67 A68 A69 A70 A71 A72 A73 A74 A75 A76 A77 A78 A79 A80 A81 A82 A17 A11 A6 | A11 A6 A215 A214 A213 A212 A211 A210 A209 A208 A207 A206 A205 A204 A113 A114 A115 A116 | A17 A182 A181 A180 | A16 A108 A107 A105 A18 A317 A316 A315 A10 | A10 A17 A108 A16 | A311 A312 A313 A18 | A18 A313 A314 A315 A10 A317 A318 A277 A278 A279 A280 A281 A282 A283 A284 A285 A286 A287 A288 A289 A290 A291 A292 A293 A294 A295 A296 A297 A298 A299 A300 A301 A302 A303 A304 A305 A306 A307 A308 A309 A310 A311 | A10 A318 A319 A103 A320 A273 A274 A275 A100 A99 A276 A277 | A96 A97 A16 | A16 A97 A98 A99 A18 A225 A226 A228 A229 A230 A231 A232 A89 A90 A91 A233 A92 A93 A94 A95 A96 | A89 A234 A235 | A17 A224 A223 A222 A221 A220 A6 A11 | A18 A226 A227 A228 | A24 L31 L24 L25 L26 L3 L10 A14 L8 L12 L11 L14 L15 L7 L13 A10 | A10 A24 A49 A48 A47 A46 A45 A44 A43 A42 A41 A40 A39 A38 A37 A36 A35 A34 A33 A32 A31 A150 A149 A148 A147 | A147 A24 A49 A50 A23 | A18 A315 A10 | A10 A315 A314 A313 A18 | A108 A17 A224 A225 A18 A16 A105 A106 A107 | A16 A107 A108 | A318 A317 A10 | A10 A317 A18 A105 A104 A103 A319 A318 | A16 A99 A98 A97 | A234 A233 A91 A232 A89 | A23 A52 A51 A50 A49 A24 A10 | A10 A24 L3 A23 | A17 A108 A109 A110 A111 A112 A113 A204 A205 A206 A207 A208 A209 A210 A211 A212 A213 A214 A215 A6 A216 A217 A218 A220 A221 A222 A223 A224 | A226 A225 A18 | A147 A148 A149 A150 A31 A32 A33 A34 A35 A36 A37 A38 A39 A40 A41 A42 A43 A44 A45 A46 A47 A48 A49 A24 | A23 A51 A50 | L1 L2 A23 L26 L23 L24 L32 | A315 A18 A317 A10 | A315 A316 A317 A18 | A107 A106 A105 A16 | A99 A275 A100 A101 A102 A103 A320 A319 A104 A105 A18 A16 | A232 A91 A90 A89 | A23 A51 A52 | A6 A218 A217 A216 | A16 A18 A105 | A319 A320 A103 | A99 A100 A275 | A91 A233 A232 | L13 L7 L15 L14 L3 L20 A26 L19 A25 | A23 L3 L18 L17 L16 | L16 A24 L3 A23 | L2 L3 A23 | A23 L3 A24 L26 | A103 A102 A101 A100 A275 A274 A273 A320 | A25 L19 A26 L20 L3 | L16 L3 A24 | L3 L11 L12 L8 A14 L10 | A3 | A19 | A20 | L22 A28 L21 A27 | A151 picked at (24.5137, -4.0777)
extrude "Extrusion2" add sketch "Sketch1" against normal blind 3.1 contours A2 A11 A10 A18 L3 L0 | A2 A253 A252 A251 A250 A249 A248 A247 A246 A245 A244 A243 A242 A241 A240 A239 A238 A237 A236 A10 A11 | A11 A18 A178 A177 A176 A175 A174 A173 A172 A171 A170 A169 A168 A167 A166 A165 A164 A163 A162 A161 A160 A159 A158 A157 A156 A155 A154 A153 A152 A2 | A2 A152 A153 A154 A155 A156 A157 A158 A159 A160 A161 A162 A163 A164 A165 A166 A167 A168 A169 A170 A171 A172 A173 A174 A175 A176 A177 A178 A18 A16 A10 A236 A237 A238 A239 A240 A241 A242 A243 A244 A245 A246 A247 A248 A249 A250 A251 A252 A253 | A18 L0 A17 A11 | A11 A17 A178 A18 | A11 A88 A87 A86 A85 A84 A83 A18 A10 | A10 A236 A235 A89 A88 A11 | A17 L1 L31 A23 A10 A11 | A11 A10 A201 A200 A199 A198 A197 A196 A195 A194 A193 A192 A191 A190 A189 A188 A187 A186 A185 A184 A183 A182 A17 A180 A179 A178 | A178 A17 A180 A181 A182 A10 A16 A18 | A10 A16 A96 A95 A94 A93 A92 A91 A233 A234 A89 A235 A236 | A18 A83 A82 A17 A10 | A10 A17 L3 A18 | A88 A89 A235 A234 A232 A231 A230 A229 A228 A18 A11 | A11 A18 A83 A84 A85 A86 A87 A88 | A11 A116 A115 A114 A113 A204 A203 A202 A201 A10 | A10 A23 A147 A146 A145 A144 A143 A142 A141 A140 A139 A138 A137 A136 A135 A134 A133 A132 A131 A130 A129 A128 A127 A126 A125 A124 A123 A122 A121 A120 A119 A118 A117 A116 A11 | A178 A179 A180 A17 | A17 L0 L1 | A17 A82 A81 A80 A79 A78 A77 A76 A75 A74 A73 A72 A71 A70 A69 A68 A67 A66 A65 A64 A63 A62 A61 A60 A59 A58 A57 A56 A55 A54 A53 A52 A23 A10 | A10 A23 L3 A17 | A18 A11 A17 A82 A83 | A18 A228 A227 A226 A225 A224 A17 A11 | A23 L31 A24 A10 | A10 A24 A147 A23 | A201 A202 A203 A204 A113 A112 A111 A110 A109 A108 A17 A10 | A10 A17 A182 A183 A184 A185 A186 A187 A188 A189 A190 A191 A192 A193 A194 A195 A196 A197 A198 A199 A200 A201 | A116 A117 A118 A119 A120 A121 A122 A123 A124 A125 A126 A127 A128 A129 A130 A131 A132 A133 A134 A135 A136 A137 A138 A139 A140 A141 A142 A143 A144 A145 A146 A147 A23 A50 A51 A52 A53 A54 A55 A56 A57 A58 A59 A60 A61 A62 A63 A64 A65 A66 A67 A68 A69 A70 A71 A72 A73 A74 A75 A76 A77 A78 A79 A80 A81 A82 A17 A11 A6 | A11 A6 A215 A214 A213 A212 A211 A210 A209 A208 A207 A206 A205 A204 A113 A114 A115 A116 | A17 A182 A181 A180 | A10 A17 A108 A16 | A16 A97 A98 A99 A18 A225 A226 A228 A229 A230 A231 A232 A89 A90 A91 A233 A92 A93 A94 A95 A96 | A89 A234 A235 | A17 A224 A223 A222 A221 A220 A6 A11 | A18 A226 A227 A228 | A24 L31 L24 L25 L26 L3 L10 A14 L8 L12 L11 L14 L15 L7 L13 A10 | A10 A24 A49 A48 A47 A46 A45 A44 A43 A42 A41 A40 A39 A38 A37 A36 A35 A34 A33 A32 A31 A150 A149 A148 A147 | A147 A24 A49 A50 A23 | A108 A17 A224 A225 A18 A16 A105 A106 A107 | A16 A99 A98 A97 | A234 A233 A91 A232 A89 | A23 A52 A51 A50 A49 A24 A10 | A10 A24 L3 A23 | A17 A108 A109 A110 A111 A112 A113 A204 A205 A206 A207 A208 A209 A210 A211 A212 A213 A214 A215 A6 A216 A217 A218 A220 A221 A222 A223 A224 | A226 A225 A18 | A147 A148 A149 A150 A31 A32 A33 A34 A35 A36 A37 A38 A39 A40 A41 A42 A43 A44 A45 A46 A47 A48 A49 A24 | A23 A51 A50 | L1 L2 A23 L26 L23 L24 L32 | A107 A106 A105 A16 | A232 A91 A90 A89 | A23 A51 A52 | A6 A218 A217 A216 | A91 A233 A232 | L13 L7 L15 L14 L3 L20 A26 L19 A25 | A23 L3 L18 L17 L16 | L16 A24 L3 A23 | L2 L3 A23 | A23 L3 A24 L26 | A25 L19 A26 L20 L3 | L16 L3 A24 | L3 L11 L12 L8 A14 L10 | A3 | A19 | A20 | L22 A28 L21 A27 picked at (24.5137, -4.0777)
extrude "Extrusion3" add sketch "Sketch1" against normal blind 6.2 contours A2 A11 A10 A18 L3 L0 | A2 A253 A252 A251 A250 A249 A248 A247 A246 A245 A244 A243 A242 A241 A240 A239 A238 A237 A236 A10 A11 | A11 A18 A178 A177 A176 A175 A174 A173 A172 A171 A170 A169 A168 A167 A166 A165 A164 A163 A162 A161 A160 A159 A158 A157 A156 A155 A154 A153 A152 A2 | A2 A152 A153 A154 A155 A156 A157 A158 A159 A160 A161 A162 A163 A164 A165 A166 A167 A168 A169 A170 A171 A172 A173 A174 A175 A176 A177 A178 A18 A16 A10 A236 A237 A238 A239 A240 A241 A242 A243 A244 A245 A246 A247 A248 A249 A250 A251 A252 A253 | A18 L0 A17 A11 | A11 A17 A178 A18 | A17 L1 L31 A23 A10 A11 | A11 A10 A201 A200 A199 A198 A197 A196 A195 A194 A193 A192 A191 A190 A189 A188 A187 A186 A185 A184 A183 A182 A17 A180 A179 A178 | A178 A17 A180 A181 A182 A10 A16 A18 | A10 A17 L3 A18 | A178 A179 A180 A17 | A17 L0 L1 | A10 A23 L3 A17 | A23 L31 A24 A10 | A10 A17 A182 A183 A184 A185 A186 A187 A188 A189 A190 A191 A192 A193 A194 A195 A196 A197 A198 A199 A200 A201 | A17 A182 A181 A180 | A24 L31 L24 L25 L26 L3 L10 A14 L8 L12 L11 L14 L15 L7 L13 A10 | A10 A24 L3 A23 | L1 L2 A23 L26 L23 L24 L32 | L13 L7 L15 L14 L3 L20 A26 L19 A25 | A23 L3 L18 L17 L16 | L16 A24 L3 A23 | L2 L3 A23 | A23 L3 A24 L26 | A25 L19 A26 L20 L3 | L16 L3 A24 | L3 L11 L12 L8 A14 L10 | A3 | A19 | A20 | L22 A28 L21 A27 picked at (24.5137, -4.0777)
ref_plane "Work Plane1" through (6.5814, -41.0408, -9.3) normal (0, 0, -1) x (0.0707652, 0.997493, 0)
extrude "Extrusion4" add sketch "Sketch1" against normal up to surface (9.3 mm away) contours A2 A11 A10 A18 L3 L0 | A18 L0 A17 A11 | A17 L1 L31 A23 A10 A11 | A10 A17 L3 A18 | A17 L0 L1 | A10 A23 L3 A17 | A23 L31 A24 A10 | A24 L31 L24 L25 L26 L3 L10 A14 L8 L12 L11 L14 L15 L7 L13 A10 | A10 A24 L3 A23 | L1 L2 A23 L26 L23 L24 L32 | L13 L7 L15 L14 L3 L20 A26 L19 A25 | A23 L3 L18 L17 L16 | L16 A24 L3 A23 | L2 L3 A23 | A23 L3 A24 L26 | A25 L19 A26 L20 L3 | L16 L3 A24 | L3 L11 L12 L8 A14 L10 | A3 | A19 | A20 | L22 A28 L21 A27 picked at (24.5137, -4.0777)
sketch "Sketch2" plane through (0, 0, 0) normal (0, 0, 1) x (1, 0, 0)
  line L0 (23.1, 0) -> (0, 0)
  line L1 (0, 0) -> (0, -29.4)
  line L2 (0, -29.4) -> (23.1, -29.4)
  line L3 (23.1, -29.4) -> (23.1, 0)
  arc A0 (7.8075, -4.272) -> (4.272, -7.8075) centre (14.7, -14.7) ccw
  line L4 (4.272, -7.8075) -> (8.6896, -12.2251)
  arc A1 (12.2251, -8.6896) -> (8.6896, -12.2251) centre (14.7, -14.7) ccw construction
  line L5 (12.2251, -8.6896) -> (7.8075, -4.272)
  line L6 (20.7104, -17.1749) -> (25.128, -21.5925)
  arc A2 (21.5925, -25.128) -> (25.128, -21.5925) centre (14.7, -14.7) ccw
  line L7 (21.5925, -25.128) -> (17.1749, -20.7104)
  line L8 (7.8075, -4.272) -> (23.1, -4.272)
  line L9 (12.2251, -8.6896) -> (8.6896, -12.2251)
  line L10 (12.2251, -8.6896) -> (23.1, -8.6896)
  line L11 (20.7104, -17.1749) -> (23.1, -17.1749)
  line L12 (20.7104, -17.1749) -> (17.1749, -20.7104)
  line L13 (21.5925, -25.128) -> (23.1, -25.128)
  line L14 (18.8355, -20.9568) -> (21.7016, -23.8229) projected
  arc A3 (21.7016, -23.8229) -> (23.8229, -21.7016) centre (14.7, -14.7) ccw projected
  line L15 (23.8229, -21.7016) -> (20.9568, -18.8355) projected
  arc A4 (18.8355, -20.9568) -> (20.9568, -18.8355) centre (14.7, -14.7) ccw projected
  arc A5 (7.6984, -5.5771) -> (5.5771, -7.6984) centre (14.7, -14.7) ccw projected
  line L16 (5.5771, -7.6984) -> (8.4432, -10.5645) projected
  arc A6 (10.5645, -8.4432) -> (8.4432, -10.5645) centre (14.7, -14.7) ccw projected
  line L17 (10.5645, -8.4432) -> (7.6984, -5.5771) projected
  circle A7 centre (14.7, -14.7) radius 5 projected
  circle A8 centre (14.7, -14.7) radius 14 projected
  circle A9 centre (14.7, -14.7) radius 14.7 projected
  circle A10 centre (14.7, -14.7) radius 14 projected
  circle A11 centre (14.7, -14.7) radius 5
  arc A12 (17.1749, -20.7104) -> (20.7104, -17.1749) centre (14.7, -14.7) ccw construction
  point P0 (0, 0)
  point P1 (23.1, -23.9569)
  point P2 (23.1, -19.5645)
  point P3 (20.0033, -20.0033)
  dimension "d34" = 6.3
  dimension "d35" = 1
  dimension "d36" = 1
  dimension "d39" = 1
  dimension "d41" = 1
  dimension "d50" = 1
  dimension "d51" = 1
  dimension "d53" = 1
  dimension "d55" = 1
  constraints: 28 end point, 9 point on circle, 5 centre point, 5 coincident, 5 perpendicular, 5 point on line, 4 tangent, 3 parallel, 1 horizontal
  measures "d34" distance edge to line of A9 L3
  measures "d35" distance between parallel lines of L4 L16
  measures "d36" distance between parallel lines of L5 L17
  measures "d39" distance between parallel lines of L7 L14
  measures "d41" distance between parallel lines of L6 L15
  measures "d50" radial gap between concentric circles of A1 A6
  measures "d51" radial gap between concentric circles of A5 A0
  measures "d53" radial gap between concentric circles of A3 A2
  measures "d55" radial gap between concentric circles of A4 A12
extrude "Extrusion5" cut sketch "Sketch2" against normal blind 3 contours L3 L10 L5 L8 | L5 L9 L4 A0 | L3 L6 L11 | A2 L7 L12 L6 L3 L15 A4 L14 A3 | A3 L14 A4 L15 L3 | L17 A6 L16 A5 | A7
sketch "Sketch3" plane through (27.4, 0, -9.3) normal (0, 0, -1) x (-1, 0, 0)
  circle A0 centre (18.3569, -61.2939) radius 1.0564
  circle A1 centre (7.0431, -49.9802) radius 1.0564
  circle A2 centre (12.7, -55.6371) radius 14.7
  circle A3 centre (12.7, -14.7) radius 14.7
  line L0 (4.3, -65.8371) -> (27.4, -65.8371)
  line L1 (27.4, -65.8371) -> (27.4, 0)
  line L2 (27.4, 0) -> (4.3, 0)
  line L3 (0, -4.272) -> (0, 0)
  line L4 (0, -4.272) -> (0, 0) projected
  line L5 (0, 0) -> (27.4, 0) projected
  line L6 (4.3, 0) -> (0, 0)
  line L7 (25.9, -1) -> (25.9, -17)
  line L8 (24.9, -1) -> (25.9, -1)
  line L9 (24.9, -17) -> (24.9, -1)
  line L10 (24.9, -17) -> (25.9, -17)
  line L11 (27.4, -19.5) -> (4.3, -19.5)
  line L12 (4.3, -19.5) -> (4.3, -23.9569)
  line L13 (4.3, -19.5) -> (0, -19.5)
  line L14 (0, -19.5) -> (0, -4.272) construction
  line L15 (0, -19.5) -> (0, -13.5)
  line L16 (0, -13.5) -> (24.4, -13.5)
  line L17 (24.4, -13.5) -> (24.4, -17.5)
  line L18 (24.4, -17.5) -> (26.4, -17.5)
  line L19 (26.4, -17.5) -> (26.4, -15)
  line L20 (26.4, -15) -> (27.4, -15)
  line L21 (27.4, -3.5) -> (26.4, -3.5)
  line L22 (26.4, -3.5) -> (26.4, -1)
  line L23 (26.4, -1) -> (24.4, -1)
  line L24 (24.4, -1) -> (24.4, -4.272)
  line L25 (4.3, -4.272) -> (0, -4.272) projected
  line L26 (24.4, -4.272) -> (0, -4.272)
  circle A4 centre (7.0431, -49.9802) radius 2.25
  circle A5 centre (18.3569, -61.2939) radius 2.25
  line L27 (25.9, -1) -> (25.9, -17) projected
  line L28 (24.9, -1) -> (25.9, -1) projected
  line L29 (24.9, -17) -> (24.9, -1) projected
  line L30 (24.9, -17) -> (25.9, -17) projected
  circle A6 centre (12.7, -14.7) radius 14.7 projected
  circle A7 centre (12.7, -14.7) radius 14 projected
  circle A8 centre (12.7, -55.6371) radius 14.7 projected
  circle A9 centre (12.7, -55.6371) radius 14 projected
  circle A10 centre (18.3569, -61.2939) radius 1.0564 projected
  circle A11 centre (7.0431, -49.9802) radius 1.0564 projected
  circle A12 centre (12.7, -55.6371) radius 5 projected
  circle A13 centre (12.7, -55.6371) radius 14 projected
  point P0 (24.9, -1)
  point P1 (25.9, -1)
  dimension "d81" = 4.5
  dimension "d83" = 2.5
  dimension "d84" = 6
  dimension "d85" = 0.5
  dimension "d86" = 2.5
  dimension "d87" = 0.5
  dimension "d88" = 0.5
  dimension "d89" = 2.5
  dimension "d90" = 0.5
  dimension "d91" = 0
  dimension "d92" = 0.5
  dimension "d95" = 4.5
  dimension "d96" = 4.5
  constraints: 49 end point, 8 perpendicular, 6 centre point, 6 coincident, 5 point on line, 5 tangent, 4 horizontal, 3 vertical, 1 collinear, 1 parallel
  measures "d81" distance edge to line of A2 L0
  measures "d83" distance between parallel lines of L11 L10
  measures "d84" distance between parallel lines of L11 L16
  measures "d85" distance between parallel lines of L19 L7
  measures "d86" distance between parallel lines of L18 L20
  measures "d87" distance between parallel lines of L18 L10
  measures "d88" distance between parallel lines of L9 L17
  measures "d89" distance between parallel lines of L23 L21
  measures "d90" distance between parallel lines of L7 L22
  measures "d91" distance between parallel lines of L23 L8
  measures "d92" distance between parallel lines of L9 L24
  measures "d95" diameter of A4
  measures "d96" diameter of A5
ref_plane "Work Plane3" through (1, -19, -16) normal (0, 0, 1) x (1, 0, 0)
extrude "Extrusion8" add sketch "Sketch3" along normal up to surface (6.7 mm away) contours L20 L1 L11 A3 | A3 L11 A7 L20 | L21 L22 L23 L8 L24 L26 A3 L2 L1 | A7 L11 L13 L15 L16 L17 L18 L19 L20 | L26 A7 L25 A3 | L25 L3 L5 L2 A3 | L26 L25 A7
extrude "Extrusion9" cut sketch "Sketch3" against normal blind 5.3 contours A0 | A1 | A4 | A5
ref_plane "Work Plane4" through (-5.099, -75.4361, 0) normal (0, 0, -1) x (0.7071068, 0.7071068, 0)
extrude "Extrusion10" cut sketch "Sketch3" against normal up to surface (9.3 mm away) contours A0 | A1
chamfer "Chamfer1" distance 0.5 angle 45 2 edges at (1, -3.5, -8) (1, -15, -8)
body "Solid1"
